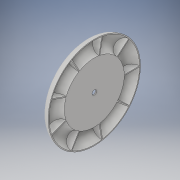
# Autodesk Inventor part: Tor
Saved by Autodesk Inventor 2019 (Build 230136000, 136)
## iProperties
Created: 2021-01-17
Part Number: Tor
Material: Типовые
Document SubType Name: Modeling
Designer: Dazer
Density: 1 g/cm^3
Appearance: По умолчанию
Author: Dazer
## iProperties of the stored document Tor_3DПЕЧАТЬ.ipt
Created: 2021-01-18
Part Number: Tor_3DПЕЧАТЬ
Material: Типовые
Document SubType Name: Modeling
Designer: Dazer
Density: 1 g/cm^3
Appearance: По умолчанию
Author: Dazer
Autodesk Inventor part; units mm, degrees
ref_plane "YZ Plane" through (0, 0, 0) normal (1, 0, 0) x (0, 1, 0)
ref_plane "XZ Plane" through (0, 0, 0) normal (0, 1, 0) x (-1, 0, 0)
ref_plane "XY Plane" through (0, 0, 0) normal (0, 0, 1) x (1, 0, 0)
sketch "Эскиз1" plane through (0, 0, 0) normal (0, 1, 0) x (-1, 0, 0)
  line L0 (0, 0) -> (3, 0)
  line L1 (0, -3.5) -> (1.4, -3.5)
  arc A0 (0, -70) -> (1.4, -44.0756) centre (0, -57) ccw
  arc A1 (0, -68.6) -> (0, -45.4) centre (0, -57) ccw
  line L2 (1.4, -3.5) -> (1.4, -44.0756)
  line L3 (0, -3.5) -> (0, -44)
  line L4 (0, -44) -> (0, -45.4)
  line L5 (0, -68.6) -> (0, -70)
  dimension "d6" = 3
  constraints: 12 end point, 4 point on circle, 3 vertical, 2 centre point, 2 point on line, 1 horizontal
  measures "d6" distance of L0.start L0.end
revolve "Вращение1" add sketch "Эскиз1" angle 360 about axis through (0, 0, 0) along (-1, 0, 0)
sketch "Эскиз2" plane through (0, 0, 0) normal (1, 0, 0) x (0, 0, -1)
  line L0 (69.3, 0) -> (69.3, 0.7)
  line L1 (69.3, 0) -> (69.3, -0.7)
  line L2 (44.7, 0) -> (44.7, -0.7)
  line L3 (44.7, -0.7) -> (69.3, -0.7)
  line L4 (44.7, 0) -> (44.7, 0.7)
  line L5 (44.7, 0.7) -> (69.3, 0.7)
  point P0 (0, 0)
  dimension "d14" = 0.7
  dimension "d15" = 0.7
  dimension "d17" = 0.7
  dimension "d18" = 0.7
  constraints: 12 end point, 1 perpendicular, 1 point on line, 1 vertical
  measures "d14" distance of L0.start L0.end
  measures "d15" distance of L0.start L1.end
  measures "d17" distance of L2.start L2.end
  measures "d18" distance of L2.start L4.end
extrude "Выдавливание1" add sketch "Эскиз2" against normal through all
pattern_circular "Круговой массив1" count 9 over 360 about axis through (-0.7, 0, 0) along (1, 0, 0) of "Выдавливание1"
